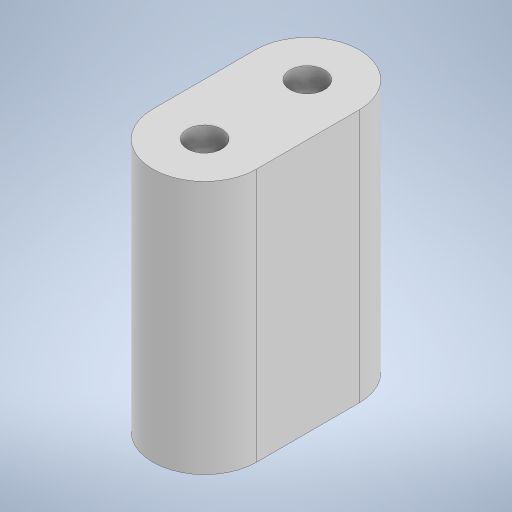
# Autodesk Inventor part: Reworked - PlateSpacers22mm
Saved by Autodesk Inventor 2023 (Build 270158000, 158)
## iProperties
Created: 2022-12-05
Part Number: Reworked - PlateSpacers22mm
Material: Generic
Document SubType Name: Modeling
Designer: Administrator
Density: 1 g/cm^3
Appearance: Default
Author: Administrator
Autodesk Inventor part; units mm, degrees
ref_plane "YZ Plane" through (0, 0, 0) normal (1, 0, 0) x (0, 1, 0)
ref_plane "XZ Plane" through (0, 0, 0) normal (0, 1, 0) x (-1, 0, 0)
ref_plane "XY Plane" through (0, 0, 0) normal (0, 0, 1) x (1, 0, 0)
sketch "Sketch1" plane through (0, 0, 0) normal (0, 1, 0) x (-1, 0, 0)
  circle A0 centre (0, 0) radius 1.5
  line L0 (0, 0) -> (0, -8.9) construction
  circle A1 centre (0, -8.9) radius 1.5
  arc A2 (-0.669, -4.45) -> (0.669, -4.45) centre (0, 0) ccw construction
  arc A3 (-4.5, -8.9) -> (4.5, -8.9) centre (0, -8.9) ccw
  line L1 (4.5, 0) -> (4.5, -8.9)
  line L2 (-4.5, -8.9) -> (-4.5, 0)
  arc A4 (-4.5, 0) -> (-0.669, -4.45) centre (0, 0) ccw construction
  arc A5 (-0.669, -4.45) -> (-4.5, -8.9) centre (0, -8.9) ccw construction
  arc A6 (0.669, -4.45) -> (-0.669, -4.45) centre (0, -8.9) ccw construction
  arc A7 (0.669, -4.45) -> (4.5, 0) centre (0, 0) ccw construction
  arc A8 (4.5, 0) -> (-4.5, 0) centre (0, 0) ccw
  arc A9 (4.5, -8.9) -> (0.669, -4.45) centre (0, -8.9) ccw construction
  dimension "d0" = 3
  dimension "d1" = 8.9
  dimension "d2" = 3
  dimension "d3" = 9
  dimension "d4" = 9
  constraints: 18 point on circle, 10 centre point, 6 end point, 6 tangent, 4 coincident, 1 vertical
  measures "d0" diameter of A0
  measures "d1" distance of L0.start L0.end
  measures "d2" diameter of A1
  measures "d3" diameter of A2
  measures "d4" diameter of A3
extrude "Extrusion1" add sketch "Sketch1" along normal blind 22
body "Solid1"
